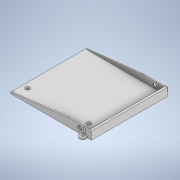
# Autodesk Inventor part: HDD
Saved by Autodesk Inventor 2020 (Build 240168000, 168)
## iProperties
Created: 2022-07-25
Part Number: HDD
Material: Типовые
Document SubType Name: Modeling
Designer: akapu
Density: 1 g/cm^3
Appearance: По умолчанию
Author: akapu
Autodesk Inventor part; units mm, degrees
ref_plane "YZ Plane" through (0, 0, 0) normal (1, 0, 0) x (0, 1, 0)
ref_plane "XZ Plane" through (0, 0, 0) normal (0, 1, 0) x (-1, 0, 0)
ref_plane "XY Plane" through (0, 0, 0) normal (0, 0, 1) x (1, 0, 0)
sketch "Эскиз1" plane through (0, 0, 0) normal (0, 1, 0) x (-1, 0, 0)
  line L0 (-3.5, 0) -> (-3.5, -76)
  line L1 (0, 0) -> (0, -2)
  line L2 (0, -2) -> (0, -1)
  line L3 (0, -72) -> (0, -73)
  line L4 (0, 0) -> (0, -12)
  line L5 (0, -12) -> (8, -12)
  line L6 (8, -12) -> (56, -12)
  line L7 (56, -12) -> (62, -12)
  line L8 (62, -12) -> (62, -1)
  line L9 (62, -1) -> (0, -1)
  line L10 (0, -73) -> (62, -73)
  line L11 (62, -73) -> (62, -12)
  line L12 (0, -72) -> (62, -72)
  line L13 (0, -2) -> (62, -2)
  line L14 (3.5, -76) -> (3.5, 0)
  line L15 (0, 0) -> (3, 0)
  line L16 (3, 0) -> (3, 0.6)
  line L17 (56, -12) -> (68, -12)
  line L18 (68, -12) -> (73, -12)
  line L19 (8, -12) -> (10, -12)
  circle A0 centre (10, -12) radius 1.1
  circle A1 centre (68, -12) radius 1.1
  circle A2 centre (3, 0.6) radius 1.1
  circle A3 centre (3, 0.6) radius 3
  circle A4 centre (4, -76) radius 1.1
  circle A5 centre (4, -76) radius 3.5
  line L20 (7.5, -76) -> (7.5, -73)
  line L21 (0.5, -76) -> (0.5, -73)
  line L22 (0, -73) -> (-3.5, -73)
  line L23 (6, 0.6) -> (6, -1)
  line L24 (0, -1) -> (-3.5, -1)
  line L25 (62, -73) -> (73, -73)
  line L26 (73, -73) -> (73, -1)
  line L27 (73, -1) -> (62, -1)
  line L28 (62, -1) -> (62, -73)
  line L29 (0, 0.6) -> (0, 0)
  point P0 (3.5, -73)
  point P1 (0.0606, 0)
  dimension "d6" = 2
  dimension "d7" = 1
  dimension "d8" = 1
  dimension "d9" = 12
  dimension "d10" = 8
  dimension "d11" = 48
  dimension "d12" = 6
  dimension "d39" = 3
  dimension "d40" = 0.6
  dimension "d41" = 12
  dimension "d42" = 5
  dimension "d43" = 2
  dimension "d44" = 2.2
  dimension "d45" = 2.2
  dimension "d46" = 2.2
  dimension "d47" = 6
  dimension "d48" = 2.2
  dimension "d49" = 7
  constraints: 60 end point, 12 perpendicular, 12 point on line, 7 coincident, 6 centre point, 4 point on circle, 4 tangent, 3 horizontal, 3 parallel, 2 collinear, 1 midpoint, 1 vertical
  measures "d6" distance of L1.start L1.end
  measures "d7" distance of L1.end L2.end
  measures "d8" distance of L3.start L3.end
  measures "d9" distance of L1.start L4.end
  measures "d10" distance of L4.end L5.end
  measures "d11" distance of L5.end L6.end
  measures "d12" distance of L6.end L7.end
  measures "d39" distance of L1.start L15.end
  measures "d40" distance of L15.end L16.end
  measures "d41" distance of L17.start L17.end
  measures "d42" distance of L17.end L18.end
  measures "d43" distance of L19.start L19.end
  measures "d44" diameter of A0
  measures "d45" diameter of A1
  measures "d46" diameter of A2
  measures "d47" diameter of A3
  measures "d48" diameter of A4
  measures "d49" diameter of A5
extrude "Выдавливание1" add sketch "Эскиз1" along normal blind 2 contours L24 L1 L4 L5 L14 L12 L3 L22 L0 | L9 A3 L13 L1 | L1 L15 A3 L9 | L3 L12 L14 A5 L10 | L29 A3 L15 | L13 A3 L14 L5 L4 | A3 L15 A2 L14 L9 | L9 L14 L13 A3 | L10 A5 L21 | A3 L9 L14 A2 L15 | L13 L14 A3 | L9 A3 L13 L14 | L14 L5 L6 A0 L7 L11 L12 | L12 L11 L10 A5 L14 | A5 L14 L10 | L10 A5 | L23 L9 A3 | L14 A3 L13 L8 L7 L6 A0 L5 | L13 A3 L14 | L9 L8 L13 A3 | L11 L17 A1 L18 L26 L25 | A5 L10 L14 | A5 L10 L20 | L8 L27 L26 L18 A1 L17
sketch "Эскиз2" plane through (0, 2, 0) normal (0, 1, 0) x (1, 0, 0)
  line L0 (-73, 1) -> (-6, 1) projected
  line L1 (3.5, 1) -> (3.5, 73) projected
  line L2 (-73, 1) -> (3.5, 1)
  line L3 (3.5, 1) -> (3.5, 2)
  line L4 (3.5, 2) -> (-73, 2)
  line L5 (-73, 2) -> (-73, 1)
  line L6 (-7.5, 73) -> (-73, 73) projected
  line L7 (-73, 73) -> (3.5, 73)
  line L8 (3.5, 73) -> (3.5, 72)
  line L9 (3.5, 72) -> (-73, 72)
  line L10 (-73, 72) -> (-73, 73)
  line L11 (0, 1) -> (3.5, 1) projected
  line L12 (3.5, 73) -> (1.5, 73)
  line L13 (1.5, 73) -> (1.5, 1)
  line L14 (1.5, 1) -> (3.5, 1)
  line L15 (3.5, 1) -> (3.5, 73)
  point P0 (-62, 73)
  point P1 (1.5, 72)
  point P2 (1.5, 2)
  dimension "d50" = 1
  dimension "d51" = 1
  dimension "d52" = 2
  constraints: 24 end point, 6 parallel, 3 horizontal, 3 perpendicular, 3 point on line
  measures "d50" distance of L3.end L2.end
  measures "d51" distance of L7.end L8.end
  measures "d52" distance of L14.end L13.end
extrude "Выдавливание2" add sketch "Эскиз2" along normal blind 6
sketch "Эскиз3" plane through (-62, 0, -1) normal (0, 0, 1) x (1, 0, 0)
  line L0 (65.5, 8) -> (-11, 8) projected
  line L1 (65.5, 8) -> (43.5, 8)
  line L2 (63.5, 8) -> (54.5, 8)
  line L3 (54.5, 8) -> (54.5, 5)
  circle A0 centre (54.5, 5) radius 1.5
  line L4 (-11, 2) -> (63.5, 2) projected
  line L5 (43.5, 8) -> (-11, 2)
  line L6 (-11, 2) -> (-11, 8)
  line L7 (43.5, 8) -> (-11, 8)
  point P0 (65.5, 2)
  dimension "d53" = 22
  dimension "d54" = 9
  dimension "d55" = 3
  dimension "d56" = 3
  constraints: 12 end point, 2 perpendicular, 1 centre point, 1 coincident, 1 collinear, 1 midpoint, 1 point on line
  measures "d53" distance of L0.start L1.end
  measures "d54" distance of L2.start L2.end
  measures "d55" distance of L2.end L3.end
  measures "d56" diameter of A0
extrude "Выдавливание3" cut sketch "Эскиз3" against normal blind 76
sketch "Эскиз4" plane through (0, 8, 0) normal (0, 1, 0) x (1, 0, 0)
  circle A0 centre (-3, -0.6) radius 1.1 projected
  circle A1 centre (-3, -0.6) radius 2.1
  dimension "d57" = 4.2
  constraints: 1 centre point, 1 coincident
  measures "d57" diameter of A1
extrude "Выдавливание4" cut sketch "Эскиз4" against normal blind 6 contours A0 | A1
chamfer "Фаска1" distance 1 angle 45 2 edges at (-8.9, 2, -12) (-66.9, 2, -12)
chamfer "Фаска2" distance 0.5 angle 45 2 edges at (-9, 5, -1) (-9, 5, -73)
sketch "Эскиз5" plane through (0, 0, 0) normal (0, -1, 0) x (1, 0, 0)
  line L0 (31.0823, 41.3034) -> (-105.9038, 41.3034)
  line L1 (-105.9038, 41.3034) -> (-105.9038, -112.9994)
  line L2 (-105.9038, -112.9994) -> (31.0823, -112.9994)
  line L3 (31.0823, -112.9994) -> (31.0823, 41.3034)
  point P0 (0, 0)
  constraints: 8 end point, 2 parallel, 1 horizontal, 1 perpendicular
extrude "Выдавливание5" cut sketch "Эскиз5" against normal blind 0.5
